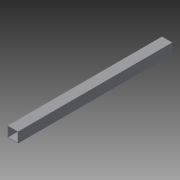
# Autodesk Inventor part: TV mount center
Saved by Autodesk Inventor 2015 (Build 190159000, 159)
## iProperties
Created: 2016-03-22
Part Number: TV mount center
Material: Generic
Document SubType Name: Modeling
Designer: Mac
Density: 1 g/cm^3
Appearance: Default
Author: Mac
Autodesk Inventor part; units mm, degrees
ref_plane "YZ Plane" through (0, 0, 0) normal (1, 0, 0) x (0, 1, 0)
ref_plane "XZ Plane" through (0, 0, 0) normal (0, 1, 0) x (-1, 0, 0)
ref_plane "XY Plane" through (0, 0, 0) normal (0, 0, 1) x (1, 0, 0)
sketch "Sketch1" plane through (0, 0, 0) normal (0, 0, 1) x (1, 0, 0)
  line L0 (-25.4, 25.4) -> (25.4, 25.4)
  line L1 (25.4, 25.4) -> (25.4, -25.4)
  line L2 (25.4, -25.4) -> (-25.4, -25.4)
  line L3 (-25.4, -25.4) -> (-25.4, 25.4)
  line L4 (23.2918, 23.2918) -> (-23.2918, 23.2918)
  line L5 (-23.2918, 23.2918) -> (-23.2918, -23.2918)
  line L6 (-23.2918, -23.2918) -> (23.2918, -23.2918)
  line L7 (23.2918, -23.2918) -> (23.2918, 23.2918)
  point P0 (0, 0)
  point P1 (0, 25.4)
  point P2 (23.2918, 0)
  dimension "d0" = 50.8
  dimension "d1" = 50.8
  dimension "d2" = 2.1082
  constraints: 16 end point, 4 parallel, 2 midpoint, 2 perpendicular, 1 horizontal, 1 horizontal alignment, 1 vertical alignment, 3 other
  measures "d0" distance of L0.start L0.end
  measures "d1" distance of L0.end L1.end
  measures "d2" distance between parallel lines of L4 L0
extrude "Extrusion1" add sketch "Sketch1" along normal mid plane 838.2
sketch "Sketch2" plane through (-25.4, 25.4, 419.1) normal (0, 1, 0) x (1, 0, 0)
  line L0 (50.8, 0) -> (109.4588, 0) construction
  line L1 (50.8, 838.2) -> (109.4588, 838.2) construction
  line L2 (50.8, 0) -> (0, 13.6118)
  line L3 (50.8, 0) -> (103.392, 0) construction
  line L4 (0, 13.6118) -> (0, 0)
  line L5 (0, 0) -> (50.8, 0)
  line L6 (50.8, 838.2) -> (109.4588, 838.2) construction
  line L7 (0, 838.2) -> (50.8, 838.2)
  line L8 (0, 838.2) -> (0, 0) projected
  line L9 (50.8, 838.2) -> (0, 824.5882)
  line L10 (50.8, 838.2) -> (103.392, 838.2) construction
  line L11 (0, 824.5882) -> (0, 838.2)
  point P0 (25.4, 419.1)
  dimension "d7" = 165
  dimension "d11" = 165
  constraints: 22 end point, 5 horizontal, 2 equal length, 2 perpendicular, 1 collinear, 1 point on line
  measures "d7" angle of L3 L2
  measures "d11" angle of L9 L10
extrude "Extrusion2" cut sketch "Sketch2" against normal through all
body "Solid1"
